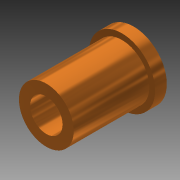
# Autodesk Inventor part: Bushing
Saved by Autodesk Inventor 2015 (Build 190159000, 159)
## iProperties
Created: 2014-12-01
Part Number: Bushing
Material: Copper, Cast
Document SubType Name: Modeling
Designer: lethcoec
Density: 8.94 g/cm^3
Appearance: Default
Author: lethcoec
Autodesk Inventor part; units mm, degrees
ref_plane "YZ Plane" through (0, 0, 0) normal (1, 0, 0) x (0, 1, 0)
ref_plane "XZ Plane" through (0, 0, 0) normal (0, 1, 0) x (-1, 0, 0)
ref_plane "XY Plane" through (0, 0, 0) normal (0, 0, 1) x (1, 0, 0)
sketch "Sketch1" plane through (0, 0, 0) normal (0, 0, 1) x (1, 0, 0)
  circle A0 centre (0, 0) radius 4.7625
  dimension "d0" = 9.525
  constraints: 1 centre point, 1 coincident
  measures "d0" diameter of A0
extrude "Extrusion1" add sketch "Sketch1" along normal blind 1.6866
sketch "Sketch2" plane through (0, 0, 1.6866) normal (0, 0, 1) x (1, 0, 0)
  circle A0 centre (0, 0) radius 4.7625 projected
  line L0 (-4.7625, 0) -> (-3.937, 0)
  circle A1 centre (0, 0) radius 3.937
  dimension "d3" = 0.8255
  constraints: 2 end point, 2 horizontal alignment, 1 coincident, 1 horizontal, 3 other
  measures "d3" distance of L0.start L0.end
extrude "Extrusion2" add sketch "Sketch2" along normal blind 10.8687 contours A1
sketch "Sketch3" plane through (0, 0, 12.5552) normal (0, 0, 1) x (1, 0, 0)
  circle A0 centre (0, 0) radius 2.3368
  dimension "d6" = 4.6736
  constraints: 1 centre point, 1 coincident
  measures "d6" diameter of A0
extrude "Extrusion3" cut sketch "Sketch3" against normal blind 31.9938
body "Solid1"
